Autodesk Fusion 360 part; units mm, degrees
(part 3 of 5)
sketch "Left Projection" plane through (0, 0, 0) normal (0, 0, 1) x (1, 0, 0) in component "Left"
  line L0 (-300.4387, -28.095) -> (-302, -28.095)
  line L1 (-302, -37.905) -> (-300.4387, -37.905)
  arc A0 (-300.4387, -37.905) -> (-298.825, -36.7758) centre (-299.5321, -37.4829) ccw
  line L2 (-298.825, -36.7758) -> (-298.825, -29.2242)
  arc A1 (-298.825, -29.2242) -> (-300.4387, -28.095) centre (-299.5321, -28.5171) ccw
  line L3 (-302, -57.905) -> (-300.4387, -57.905)
  line L4 (-300.4387, -48.095) -> (-302, -48.095)
  arc A2 (-298.825, -49.2242) -> (-300.4387, -48.095) centre (-299.5321, -48.5171) ccw
  line L5 (-298.825, -56.7758) -> (-298.825, -49.2242)
  arc A3 (-300.4387, -57.905) -> (-298.825, -56.7758) centre (-299.5321, -57.4829) ccw
  line L6 (-302, -77.905) -> (-300.4387, -77.905)
  line L7 (-300.4387, -68.095) -> (-302, -68.095)
  arc A4 (-298.825, -69.2242) -> (-300.4387, -68.095) centre (-299.5321, -68.5171) ccw
  line L8 (-298.825, -76.7758) -> (-298.825, -69.2242)
  arc A5 (-300.4387, -77.905) -> (-298.825, -76.7758) centre (-299.5321, -77.4829) ccw
  line L9 (-302, -97.905) -> (-300.4387, -97.905)
  line L10 (-300.4387, -88.095) -> (-302, -88.095)
  arc A6 (-298.825, -89.2242) -> (-300.4387, -88.095) centre (-299.5321, -88.5171) ccw
  line L11 (-298.825, -96.7758) -> (-298.825, -89.2242)
  arc A7 (-300.4387, -97.905) -> (-298.825, -96.7758) centre (-299.5321, -97.4829) ccw
  line L12 (-302, -117.905) -> (-300.4387, -117.905)
  line L13 (-300.4387, -108.095) -> (-302, -108.095)
  arc A8 (-298.825, -109.2242) -> (-300.4387, -108.095) centre (-299.5321, -108.5171) ccw
  line L14 (-298.825, -116.7758) -> (-298.825, -109.2242)
  arc A9 (-300.4387, -117.905) -> (-298.825, -116.7758) centre (-299.5321, -117.4829) ccw
  line L15 (-302, -137.905) -> (-300.4387, -137.905)
  line L16 (-300.4387, -128.095) -> (-302, -128.095)
  arc A10 (-298.825, -129.2242) -> (-300.4387, -128.095) centre (-299.5321, -128.5171) ccw
  line L17 (-298.825, -136.7758) -> (-298.825, -129.2242)
  arc A11 (-300.4387, -137.905) -> (-298.825, -136.7758) centre (-299.5321, -137.4829) ccw
  line L18 (-302, -157.905) -> (-300.4387, -157.905)
  line L19 (-300.4387, -168.095) -> (-302, -168.095)
  arc A12 (-298.825, -169.2242) -> (-300.4387, -168.095) centre (-299.5321, -168.5171) ccw
  line L20 (-298.825, -184) -> (-298.825, -169.2242)
  line L21 (-298.825, -16.7758) -> (-298.825, -2)
  arc A13 (-300.4387, -17.905) -> (-298.825, -16.7758) centre (-299.5321, -17.4829) ccw
  line L22 (-302, -17.905) -> (-300.4387, -17.905)
  line L23 (-300.4387, -148.095) -> (-302, -148.095)
  arc A14 (-298.825, -149.2242) -> (-300.4387, -148.095) centre (-299.5321, -148.5171) ccw
  line L24 (-298.825, -156.7758) -> (-298.825, -149.2242)
  arc A15 (-300.4387, -157.905) -> (-298.825, -156.7758) centre (-299.5321, -157.4829) ccw
  line L25 (-298.825, -2) -> (-286.905, -2)
  line L26 (-286.905, -2) -> (-286.905, -3.5613)
  arc A16 (-286.905, -3.5613) -> (-285.7758, -5.175) centre (-286.4829, -4.4679) ccw
  line L27 (-285.7758, -5.175) -> (-278.2242, -5.175)
  arc A17 (-278.2242, -5.175) -> (-277.095, -3.5613) centre (-277.5171, -4.4679) ccw
  line L28 (-277.095, -3.5613) -> (-277.095, -2)
  line L29 (-277.095, -2) -> (-266.905, -2)
  line L30 (-266.905, -2) -> (-266.905, -3.5613)
  arc A18 (-266.905, -3.5613) -> (-265.7758, -5.175) centre (-266.4829, -4.4679) ccw
  line L31 (-265.7758, -5.175) -> (-258.2242, -5.175)
  arc A19 (-258.2242, -5.175) -> (-257.095, -3.5613) centre (-257.5171, -4.4679) ccw
  line L32 (-257.095, -3.5613) -> (-257.095, -2)
  line L33 (-257.095, -2) -> (-245.175, -2)
  line L34 (-245.175, -2) -> (-245.175, -16.7758)
  arc A20 (-245.175, -16.7758) -> (-243.5613, -17.905) centre (-244.4679, -17.4829) ccw
  line L35 (-243.5613, -17.905) -> (-242, -17.905)
  line L36 (-242, -17.905) -> (-242, -28.095)
  line L37 (-242, -28.095) -> (-243.5613, -28.095)
  arc A21 (-243.5613, -28.095) -> (-245.175, -29.2242) centre (-244.4679, -28.5171) ccw
  line L38 (-245.175, -29.2242) -> (-245.175, -36.7758)
  arc A22 (-245.175, -36.7758) -> (-243.5613, -37.905) centre (-244.4679, -37.4829) ccw
  line L39 (-243.5613, -37.905) -> (-242, -37.905)
  line L40 (-242, -37.905) -> (-242, -48.095)
  line L41 (-243.5613, -48.095) -> (-242, -48.095)
  arc A23 (-243.5613, -48.095) -> (-245.175, -49.2242) centre (-244.4679, -48.5171) ccw
  line L42 (-245.175, -56.7758) -> (-245.175, -49.2242)
  arc A24 (-245.175, -56.7758) -> (-243.5613, -57.905) centre (-244.4679, -57.4829) ccw
  line L43 (-242, -57.905) -> (-243.5613, -57.905)
  line L44 (-242, -57.905) -> (-242, -68.095)
  line L45 (-243.5613, -68.095) -> (-242, -68.095)
  arc A25 (-243.5613, -68.095) -> (-245.175, -69.2242) centre (-244.4679, -68.5171) ccw
  line L46 (-245.175, -76.7758) -> (-245.175, -69.2242)
  arc A26 (-245.175, -76.7758) -> (-243.5613, -77.905) centre (-244.4679, -77.4829) ccw
  line L47 (-242, -77.905) -> (-243.5613, -77.905)
  line L48 (-242, -77.905) -> (-242, -88.095)
  line L49 (-243.5613, -88.095) -> (-242, -88.095)
  arc A27 (-243.5613, -88.095) -> (-245.175, -89.2242) centre (-244.4679, -88.5171) ccw
  line L50 (-245.175, -96.7758) -> (-245.175, -89.2242)
  arc A28 (-245.175, -96.7758) -> (-243.5613, -97.905) centre (-244.4679, -97.4829) ccw
  line L51 (-242, -97.905) -> (-243.5613, -97.905)
  line L52 (-242, -97.905) -> (-242, -108.095)
  line L53 (-243.5613, -108.095) -> (-242, -108.095)
  arc A29 (-243.5613, -108.095) -> (-245.175, -109.2242) centre (-244.4679, -108.5171) ccw
  line L54 (-245.175, -116.7758) -> (-245.175, -109.2242)
  arc A30 (-245.175, -116.7758) -> (-243.5613, -117.905) centre (-244.4679, -117.4829) ccw
  line L55 (-242, -117.905) -> (-243.5613, -117.905)
  line L56 (-242, -117.905) -> (-242, -128.095)
  line L57 (-243.5613, -128.095) -> (-242, -128.095)
  arc A31 (-243.5613, -128.095) -> (-245.175, -129.2242) centre (-244.4679, -128.5171) ccw
  line L58 (-245.175, -136.7758) -> (-245.175, -129.2242)
  arc A32 (-245.175, -136.7758) -> (-243.5613, -137.905) centre (-244.4679, -137.4829) ccw
  line L59 (-242, -137.905) -> (-243.5613, -137.905)
  line L60 (-242, -137.905) -> (-242, -148.095)
  line L61 (-243.5613, -148.095) -> (-242, -148.095)
  arc A33 (-243.5613, -148.095) -> (-245.175, -149.2242) centre (-244.4679, -148.5171) ccw
  line L62 (-245.175, -156.7758) -> (-245.175, -149.2242)
  arc A34 (-245.175, -156.7758) -> (-243.5613, -157.905) centre (-244.4679, -157.4829) ccw
  line L63 (-242, -157.905) -> (-243.5613, -157.905)
  line L64 (-242, -157.905) -> (-242, -168.095)
  line L65 (-243.5613, -168.095) -> (-242, -168.095)
  arc A35 (-243.5613, -168.095) -> (-245.175, -169.2242) centre (-244.4679, -168.5171) ccw
  line L66 (-245.175, -184) -> (-245.175, -169.2242)
  line L67 (-245.175, -184) -> (-257.095, -184)
  line L68 (-257.095, -182.4387) -> (-257.095, -184)
  arc A36 (-257.095, -182.4387) -> (-258.2242, -180.825) centre (-257.5171, -181.5321) ccw
  line L69 (-265.7758, -180.825) -> (-258.2242, -180.825)
  arc A37 (-265.7758, -180.825) -> (-266.905, -182.4387) centre (-266.4829, -181.5321) ccw
  line L70 (-266.905, -184) -> (-266.905, -182.4387)
  line L71 (-266.905, -184) -> (-277.095, -184)
  line L72 (-277.095, -182.4387) -> (-277.095, -184)
  arc A38 (-277.095, -182.4387) -> (-278.2242, -180.825) centre (-277.5171, -181.5321) ccw
  line L73 (-285.7758, -180.825) -> (-278.2242, -180.825)
  arc A39 (-285.7758, -180.825) -> (-286.905, -182.4387) centre (-286.4829, -181.5321) ccw
  line L74 (-286.905, -184) -> (-286.905, -182.4387)
  line L75 (-286.905, -184) -> (-298.825, -184)
  line L76 (-302, -168.095) -> (-302, -157.905)
  line L77 (-302, -148.095) -> (-302, -137.905)
  line L78 (-302, -128.095) -> (-302, -117.905)
  line L79 (-302, -108.095) -> (-302, -97.905)
  line L80 (-302, -88.095) -> (-302, -77.905)
  line L81 (-302, -68.095) -> (-302, -57.905)
  line L82 (-302, -48.095) -> (-302, -37.905)
  line L83 (-302, -28.095) -> (-302, -17.905)
move_body "Move1" [suppressed] in component "Back"
sketch "Back Projection" plane through (0, 0, 0) normal (0, 0, 1) x (1, 0, 0) in component "Back"
  line L0 (5.175, -60.591) -> (5.175, -62.226)
  line L1 (5.175, -62.226) -> (15.7758, -62.226)
  arc A0 (16.905, -63.8397) -> (15.7758, -62.226) centre (16.4829, -62.9331) ccw
  line L2 (16.905, -63.8397) -> (16.905, -65.401)
  line L3 (16.905, -65.401) -> (27.095, -65.401)
  line L4 (27.095, -65.401) -> (27.095, -63.8397)
  arc A1 (28.2242, -62.226) -> (27.095, -63.8397) centre (27.5171, -62.9331) ccw
  line L5 (28.2242, -62.226) -> (35.7758, -62.226)
  arc A2 (36.905, -63.8397) -> (35.7758, -62.226) centre (36.4829, -62.9331) ccw
  line L6 (36.905, -63.8397) -> (36.905, -65.401)
  line L7 (36.905, -65.401) -> (47.095, -65.401)
  line L8 (47.095, -65.401) -> (47.095, -63.8397)
  arc A3 (48.2242, -62.226) -> (47.095, -63.8397) centre (47.5171, -62.9331) ccw
  line L9 (48.2242, -62.226) -> (55.7758, -62.226)
  arc A4 (56.905, -63.8397) -> (55.7758, -62.226) centre (56.4829, -62.9331) ccw
  line L10 (56.905, -63.8397) -> (56.905, -65.401)
  line L11 (56.905, -65.401) -> (67.095, -65.401)
  line L12 (67.095, -65.401) -> (67.095, -63.8397)
  arc A5 (68.2242, -62.226) -> (67.095, -63.8397) centre (67.5171, -62.9331) ccw
  line L13 (68.2242, -62.226) -> (75.7758, -62.226)
  arc A6 (76.905, -63.8397) -> (75.7758, -62.226) centre (76.4829, -62.9331) ccw
  line L14 (76.905, -63.8397) -> (76.905, -65.401)
  line L15 (76.905, -65.401) -> (87.095, -65.401)
  line L16 (87.095, -65.401) -> (87.095, -63.8397)
  arc A7 (88.2242, -62.226) -> (87.095, -63.8397) centre (87.5171, -62.9331) ccw
  line L17 (88.2242, -62.226) -> (95.7758, -62.226)
  arc A8 (96.905, -63.8397) -> (95.7758, -62.226) centre (96.4829, -62.9331) ccw
  line L18 (96.905, -63.8397) -> (96.905, -65.401)
  line L19 (96.905, -65.401) -> (107.095, -65.401)
  line L20 (107.095, -65.401) -> (107.095, -63.8397)
  arc A9 (108.2242, -62.226) -> (107.095, -63.8397) centre (107.5171, -62.9331) ccw
  line L21 (108.2242, -62.226) -> (115.7758, -62.226)
  arc A10 (116.905, -63.8397) -> (115.7758, -62.226) centre (116.4829, -62.9331) ccw
  line L22 (116.905, -63.8397) -> (116.905, -65.401)
  line L23 (116.905, -65.401) -> (127.095, -65.401)
  line L24 (127.095, -65.401) -> (127.095, -63.8397)
  arc A11 (128.2242, -62.226) -> (127.095, -63.8397) centre (127.5171, -62.9331) ccw
  line L25 (128.2242, -62.226) -> (135.7758, -62.226)
  arc A12 (136.905, -63.8397) -> (135.7758, -62.226) centre (136.4829, -62.9331) ccw
  line L26 (136.905, -63.8397) -> (136.905, -65.401)
  line L27 (136.905, -65.401) -> (147.095, -65.401)
  line L28 (147.095, -65.401) -> (147.095, -63.8397)
  arc A13 (148.2242, -62.226) -> (147.095, -63.8397) centre (147.5171, -62.9331) ccw
  line L29 (148.2242, -62.226) -> (155.7758, -62.226)
  arc A14 (156.905, -63.8397) -> (155.7758, -62.226) centre (156.4829, -62.9331) ccw
  line L30 (156.905, -63.8397) -> (156.905, -65.401)
  line L31 (156.905, -65.401) -> (167.095, -65.401)
  line L32 (167.095, -65.401) -> (167.095, -63.8397)
  arc A15 (168.2242, -62.226) -> (167.095, -63.8397) centre (167.5171, -62.9331) ccw
  line L33 (168.2242, -62.226) -> (175.7758, -62.226)
  arc A16 (176.905, -63.8397) -> (175.7758, -62.226) centre (176.4829, -62.9331) ccw
  line L34 (176.905, -63.8397) -> (176.905, -65.401)
  line L35 (176.905, -65.401) -> (187.095, -65.401)
  line L36 (187.095, -65.401) -> (187.095, -63.8397)
  arc A17 (188.2242, -62.226) -> (187.095, -63.8397) centre (187.5171, -62.9331) ccw
  line L37 (188.2242, -62.226) -> (195.7758, -62.226)
  arc A18 (196.905, -63.8397) -> (195.7758, -62.226) centre (196.4829, -62.9331) ccw
  line L38 (196.905, -63.8397) -> (196.905, -65.401)
  line L39 (196.905, -65.401) -> (207.095, -65.401)
  line L40 (207.095, -65.401) -> (207.095, -63.8397)
  arc A19 (208.2242, -62.226) -> (207.095, -63.8397) centre (207.5171, -62.9331) ccw
  line L41 (208.2242, -62.226) -> (215.7758, -62.226)
  arc A20 (216.905, -63.8397) -> (215.7758, -62.226) centre (216.4829, -62.9331) ccw
  line L42 (216.905, -63.8397) -> (216.905, -65.401)
  line L43 (216.905, -65.401) -> (227.095, -65.401)
  line L44 (227.095, -65.401) -> (227.095, -63.8397)
  arc A21 (228.2242, -62.226) -> (227.095, -63.8397) centre (227.5171, -62.9331) ccw
  line L45 (228.2242, -62.226) -> (238.825, -62.226)
  line L46 (238.825, -62.226) -> (238.825, -60.591)
  arc A22 (238.825, -59.1768) -> (238.825, -60.591) centre (239.5321, -59.8839) ccw
  line L47 (238.825, -59.1768) -> (238.825, -51.6252)
  arc A23 (240.4387, -50.496) -> (238.825, -51.6252) centre (239.5321, -50.9181) ccw
  line L48 (240.4387, -50.496) -> (242, -50.496)
  line L49 (242, -50.496) -> (242, -40.306)
  line L50 (242, -40.306) -> (240.4387, -40.306)
  arc A24 (238.825, -39.1768) -> (240.4387, -40.306) centre (239.5321, -39.8839) ccw
  line L51 (238.825, -39.1768) -> (238.825, -31.6252)
  arc A25 (240.4387, -30.496) -> (238.825, -31.6252) centre (239.5321, -30.9181) ccw
  line L52 (240.4387, -30.496) -> (242, -30.496)
  line L53 (242, -30.496) -> (242, -20.306)
  line L54 (242, -20.306) -> (240.4387, -20.306)
  arc A26 (238.825, -19.1768) -> (240.4387, -20.306) centre (239.5321, -19.8839) ccw
  line L55 (238.825, -19.1768) -> (238.825, -11.6252)
  arc A27 (238.825, -10.211) -> (238.825, -11.6252) centre (239.5321, -10.9181) ccw
  line L56 (238.825, -10.211) -> (238.825, -8.576)
  line L57 (238.825, -8.576) -> (228.2242, -8.576)
  arc A28 (227.095, -6.9623) -> (228.2242, -8.576) centre (227.5171, -7.8689) ccw
  line L58 (227.095, -6.9623) -> (227.095, -5.401)
  line L59 (227.095, -5.401) -> (216.905, -5.401)
  line L60 (216.905, -5.401) -> (216.905, -6.9623)
  arc A29 (215.7758, -8.576) -> (216.905, -6.9623) centre (216.4829, -7.8689) ccw
  line L61 (215.7758, -8.576) -> (208.2242, -8.576)
  arc A30 (207.095, -6.9623) -> (208.2242, -8.576) centre (207.5171, -7.8689) ccw
  line L62 (207.095, -6.9623) -> (207.095, -5.401)
  line L63 (207.095, -5.401) -> (196.905, -5.401)
  line L64 (196.905, -5.401) -> (196.905, -6.9623)
  arc A31 (195.7758, -8.576) -> (196.905, -6.9623) centre (196.4829, -7.8689) ccw
  line L65 (195.7758, -8.576) -> (188.2242, -8.576)
  arc A32 (187.095, -6.9623) -> (188.2242, -8.576) centre (187.5171, -7.8689) ccw
  line L66 (187.095, -6.9623) -> (187.095, -5.401)
  line L67 (187.095, -5.401) -> (176.905, -5.401)
  line L68 (176.905, -5.401) -> (176.905, -6.9623)
  arc A33 (175.7758, -8.576) -> (176.905, -6.9623) centre (176.4829, -7.8689) ccw
  line L69 (175.7758, -8.576) -> (168.2242, -8.576)
  arc A34 (167.095, -6.9623) -> (168.2242, -8.576) centre (167.5171, -7.8689) ccw
  line L70 (167.095, -6.9623) -> (167.095, -5.401)
  line L71 (167.095, -5.401) -> (156.905, -5.401)
  line L72 (156.905, -5.401) -> (156.905, -6.9623)
  arc A35 (155.7758, -8.576) -> (156.905, -6.9623) centre (156.4829, -7.8689) ccw
  line L73 (155.7758, -8.576) -> (148.2242, -8.576)
  arc A36 (147.095, -6.9623) -> (148.2242, -8.576) centre (147.5171, -7.8689) ccw
  line L74 (147.095, -6.9623) -> (147.095, -5.401)
  line L75 (147.095, -5.401) -> (136.905, -5.401)
  line L76 (136.905, -5.401) -> (136.905, -6.9623)
  arc A37 (135.7758, -8.576) -> (136.905, -6.9623) centre (136.4829, -7.8689) ccw
  line L77 (135.7758, -8.576) -> (128.2242, -8.576)
  arc A38 (127.095, -6.9623) -> (128.2242, -8.576) centre (127.5171, -7.8689) ccw
  line L78 (127.095, -6.9623) -> (127.095, -5.401)
  line L79 (127.095, -5.401) -> (116.905, -5.401)
  line L80 (116.905, -5.401) -> (116.905, -6.9623)
  arc A39 (115.7758, -8.576) -> (116.905, -6.9623) centre (116.4829, -7.8689) ccw
  line L81 (115.7758, -8.576) -> (108.2242, -8.576)
  arc A40 (107.095, -6.9623) -> (108.2242, -8.576) centre (107.5171, -7.8689) ccw
  line L82 (107.095, -6.9623) -> (107.095, -5.401)
  line L83 (107.095, -5.401) -> (96.905, -5.401)
  line L84 (96.905, -5.401) -> (96.905, -6.9623)
  arc A41 (95.7758, -8.576) -> (96.905, -6.9623) centre (96.4829, -7.8689) ccw
  line L85 (95.7758, -8.576) -> (88.2242, -8.576)
  arc A42 (87.095, -6.9623) -> (88.2242, -8.576) centre (87.5171, -7.8689) ccw
  line L86 (87.095, -6.9623) -> (87.095, -5.401)
  line L87 (87.095, -5.401) -> (76.905, -5.401)
  line L88 (76.905, -5.401) -> (76.905, -6.9623)
  arc A43 (75.7758, -8.576) -> (76.905, -6.9623) centre (76.4829, -7.8689) ccw
  line L89 (75.7758, -8.576) -> (68.2242, -8.576)
  arc A44 (67.095, -6.9623) -> (68.2242, -8.576) centre (67.5171, -7.8689) ccw
  line L90 (67.095, -6.9623) -> (67.095, -5.401)
  line L91 (67.095, -5.401) -> (56.905, -5.401)
  line L92 (56.905, -5.401) -> (56.905, -6.9623)
  arc A45 (55.7758, -8.576) -> (56.905, -6.9623) centre (56.4829, -7.8689) ccw
  line L93 (55.7758, -8.576) -> (48.2242, -8.576)
  arc A46 (47.095, -6.9623) -> (48.2242, -8.576) centre (47.5171, -7.8689) ccw
  line L94 (47.095, -6.9623) -> (47.095, -5.401)
  line L95 (47.095, -5.401) -> (36.905, -5.401)
  line L96 (36.905, -5.401) -> (36.905, -6.9623)
  arc A47 (35.7758, -8.576) -> (36.905, -6.9623) centre (36.4829, -7.8689) ccw
  line L97 (35.7758, -8.576) -> (28.2242, -8.576)
  arc A48 (27.095, -6.9623) -> (28.2242, -8.576) centre (27.5171, -7.8689) ccw
  line L98 (27.095, -6.9623) -> (27.095, -5.401)
  line L99 (27.095, -5.401) -> (16.905, -5.401)
  line L100 (16.905, -5.401) -> (16.905, -6.9623)
  arc A49 (15.7758, -8.576) -> (16.905, -6.9623) centre (16.4829, -7.8689) ccw
  line L101 (15.7758, -8.576) -> (5.175, -8.576)
  line L102 (5.175, -8.576) -> (5.175, -10.211)
  arc A50 (5.175, -11.6252) -> (5.175, -10.211) centre (4.4679, -10.9181) ccw
  line L103 (5.175, -11.6252) -> (5.175, -19.1768)
  arc A51 (3.5613, -20.306) -> (5.175, -19.1768) centre (4.4679, -19.8839) ccw
  line L104 (3.5613, -20.306) -> (2, -20.306)
  line L105 (2, -20.306) -> (2, -30.496)
  line L106 (2, -30.496) -> (3.5613, -30.496)
  arc A52 (5.175, -31.6252) -> (3.5613, -30.496) centre (4.4679, -30.9181) ccw
  line L107 (5.175, -31.6252) -> (5.175, -39.1768)
  arc A53 (3.5613, -40.306) -> (5.175, -39.1768) centre (4.4679, -39.8839) ccw
  line L108 (3.5613, -40.306) -> (2, -40.306)
  line L109 (2, -40.306) -> (2, -50.496)
  line L110 (2, -50.496) -> (3.5613, -50.496)
  arc A54 (5.175, -51.6252) -> (3.5613, -50.496) centre (4.4679, -50.9181) ccw
  line L111 (5.175, -51.6252) -> (5.175, -59.1768)
  arc A55 (5.175, -60.591) -> (5.175, -59.1768) centre (4.4679, -59.8839) ccw
sketch "Plaform" plane through (0, 0, 0) normal (0, 0, 1) x (1, 0, 0) in component "Platform"
  line L0 (-255.6038, 317) -> (-88.6038, 317)
  line L1 (-85.6038, 314) -> (-85.6038, 203)
  line L2 (-88.6038, 200) -> (-255.6038, 200)
  line L3 (-258.6038, 203) -> (-258.6038, 314)
  line L4 (1.75, 0) -> (22.5, 0)
  line L5 (0, 1.75) -> (0, 22.5)
  line L6 (-178.6038, 263) -> (-165.6038, 263)
  line L7 (-163.6038, 261) -> (-163.6038, 256)
  line L8 (-165.6038, 254) -> (-178.6038, 254)
  line L9 (-180.6038, 256) -> (-180.6038, 261)
  line L10 (-187.1038, 314) -> (-157.1038, 314) construction
  line L11 (-157.1038, 314) -> (-157.1038, 203) construction
  line L12 (-157.1038, 203) -> (-187.1038, 203) construction
  line L13 (-187.1038, 203) -> (-187.1038, 314) construction
  line L14 (-187.1038, 314) -> (-157.1038, 203) construction
  line L15 (-157.1038, 314) -> (-187.1038, 203) construction
  circle A0 centre (-187.1038, 314) radius 1.5
  circle A1 centre (-157.1038, 314) radius 1.5
  circle A2 centre (-157.1038, 203) radius 1.5
  circle A3 centre (-187.1038, 203) radius 1.5
  line L16 (-239.1038, 305) -> (-105.1038, 305) construction
  line L17 (-105.1038, 212) -> (-239.1038, 212) construction
  line L18 (-239.1038, 212) -> (-239.1038, 305) construction
  line L19 (-239.1038, 305) -> (-105.1038, 212) construction
  line L20 (-105.1038, 305) -> (-239.1038, 212) construction
  line L21 (-89.1038, 203.5) -> (-255.1038, 203.5) construction
  line L22 (-255.1038, 203.5) -> (-255.1038, 313.5) construction
  line L23 (-255.1038, 313.5) -> (-89.1038, 313.5) construction
  line L24 (-89.1038, 203.5) -> (-255.1038, 313.5) construction
  line L25 (-255.1038, 203.5) -> (-89.1038, 313.5) construction
  circle A4 centre (-255.1038, 203.5) radius 1.75
  circle A5 centre (-255.1038, 313.5) radius 1.75
  circle A6 centre (-89.1038, 313.5) radius 1.75
  circle A7 centre (-89.1038, 203.5) radius 1.75
  circle A8 centre (-118.6038, 258.5) radius 1.5
  circle A9 centre (-88.6038, 258.5) radius 1.5
  arc A10 (-88.6038, 200) -> (-85.6038, 203) centre (-88.6038, 203) ccw
  arc A11 (-258.6038, 203) -> (-255.6038, 200) centre (-255.6038, 203) ccw
  arc A12 (-255.6038, 317) -> (-258.6038, 314) centre (-255.6038, 314) ccw
  arc A13 (-85.6038, 314) -> (-88.6038, 317) centre (-88.6038, 314) ccw
  circle A14 centre (-239.1038, 305) radius 1.75
  circle A15 centre (-105.1038, 305) radius 1.75
  circle A16 centre (-105.1038, 212) radius 1.75
  circle A17 centre (-239.1038, 212) radius 1.75
  line L26 (-105.1038, 305) -> (-105.1038, 212) construction
  arc A18 (-178.6038, 263) -> (-180.6038, 261) centre (-178.6038, 261) ccw
  arc A19 (-163.6038, 261) -> (-165.6038, 263) centre (-165.6038, 261) ccw
  arc A20 (-180.6038, 256) -> (-178.6038, 254) centre (-178.6038, 256) ccw
  arc A21 (-165.6038, 254) -> (-163.6038, 256) centre (-165.6038, 256) ccw
  point P0 (-258.6038, 317)
  point P1 (-85.6038, 317)
  point P2 (-258.6038, 200)
  point P3 (-180.6038, 263)
  point P4 (-163.6038, 263)
  point P5 (-180.6038, 254)
  point P6 (-85.6038, 258.5)
  point P7 (-172.1038, 263)
  point P8 (-172.1038, 317)
  point P9 (-172.1038, 258.5)
  point P10 (-172.1038, 258.5)
  point P11 (-172.1038, 258.5)
  point P12 (-258.6038, 258.5)
  point P13 (-172.1038, 200)
  point P14 (-255.1038, 258.5)
  point P15 (-180.6038, 258.5)
  point P16 (-172.1038, 254)
  dimension "d1498" = 173
  dimension "d1499" = 117
  dimension "d1500" = 200
  dimension "d1501" = 85.6038
  dimension "d1502" = 17
  dimension "d1503" = 9
  dimension "d1505" = 30
  dimension "d1506" = 111
  dimension "d1507" = 3
  dimension "d1508" = 3
  dimension "d1509" = 3
  dimension "d1510" = 3
  dimension "d1512" = 93
  dimension "d1513" = 166
  dimension "d1514" = 110
  dimension "d1515" = 3.5
  dimension "d1516" = 3.5
  dimension "d1517" = 3.5
  dimension "d1518" = 3.5
  dimension "d1552" = 3
  dimension "d1553" = 3
  dimension "d1554" = 3
  dimension "d1555" = 3
  dimension "d1557" = 3.5
  dimension "d1558" = 3.5
  dimension "d1559" = 3.5
  dimension "d1560" = 3.5
  dimension "d1611" = 3
  dimension "d1612" = 3
  dimension "d1613" = 3
  dimension "d1614" = 30
  dimension "d1615" = 134
  dimension "d1650" = 2
  dimension "d1651" = 2
  dimension "d1652" = 2
  dimension "d1653" = 2
  dimension "d1736" = 9
  constraint horizontal L0
  constraint vertical L1
  constraint horizontal L2
  constraint vertical L3
  constraint horizontal L6
  constraint vertical L7
  constraint horizontal L8
  constraint vertical L9
  constraint vertical P7 P8
  constraint horizontal L10
  constraint perpendicular L10 L11
  constraint parallel L10 L12
  constraint parallel L11 L13
  constraint coincident L14 P11
  constraint coincident L15 P11
  constraint horizontal P6 P10
  constraint vertical P8 P11
  constraint coincident L10.start L13.end
  constraint coincident L10.end L11.start
  constraint coincident L11.end L12.start
  constraint coincident L12.end L13.start
  constraint horizontal L16
  constraint parallel L16 L17
  constraint coincident L19 P11
  constraint coincident L20 P11
  constraint coincident P11 P10
  constraint horizontal L21
  constraint perpendicular L21 L22
  constraint parallel L21 L23
  constraint coincident L24 P11
  constraint coincident L25 P11
  constraint coincident L21.end L22.start
  constraint coincident L22.end L23.start
  constraint coincident L23.end L25.end
  constraint coincident L21.start L24.start
  constraint coincident L1 P6
  constraint tangent L2 A10
  constraint tangent L1 A10
  constraint coincident P2 L2
  constraint coincident P2 L3
  constraint tangent L2 A11
  constraint tangent L3 A11
  constraint coincident L0 P8
  constraint coincident P0 L3
  constraint coincident P0 L0
  constraint tangent L3 A12
  constraint tangent L0 A12
  constraint midpoint L3 P12
  constraint horizontal P11 P12
  constraint midpoint L2 P13
  constraint vertical P11 P13
  constraint coincident P1 L0
  constraint coincident P1 L1
  constraint tangent L0 A13
  constraint tangent L1 A13
  constraint coincident L16.start L18.end
  constraint coincident L16.end L20.start
  constraint coincident L17.start L19.end
  constraint coincident L17.end L18.start
  constraint perpendicular L17 L26
  constraint perpendicular L17 L18
  constraint horizontal A8.centre A9.centre
  constraint horizontal P6 A9.centre
  constraint midpoint L22 P14
  constraint horizontal P12 P14
  constraint coincident L6 P7
  constraint coincident P3 L9
  constraint coincident P3 L6
  constraint tangent L9 A18
  constraint tangent L6 A18
  constraint coincident P4 L6
  constraint coincident P4 L7
  constraint tangent L6 A19
  constraint tangent L7 A19
  constraint coincident P5 L9
  constraint coincident P5 L8
  constraint tangent L9 A20
  constraint tangent L8 A20
  constraint tangent L8 A21
  constraint tangent L7 A21
  constraint midpoint L9 P15
  constraint horizontal P11 P15
  constraint midpoint L8 P16
  constraint vertical P11 P16
  measures "d1498" distance of P0 P1
  measures "d1499" distance of P0 P2
  measures "d1500" distance of L2 L4
  measures "d1501" distance of L1 L5
  measures "d1502" distance of P3 P4
  measures "d1503" distance of P3 P5
  measures "d1505" distance of L11.end L12.end
  measures "d1506" distance of L10.start L12.end
  measures "d1507" diameter of A0
  measures "d1508" diameter of A1
  measures "d1509" diameter of A2
  measures "d1510" diameter of A3
  measures "d1512" distance of L16 L17
  measures "d1513" distance of L22.end L23.end
  measures "d1514" distance of L21.end L22.end
  measures "d1515" diameter of A4
  measures "d1516" diameter of A5
  measures "d1517" diameter of A6
  measures "d1518" diameter of A7
  measures "d1552" radius of A10
  measures "d1553" radius of A11
  measures "d1554" radius of A12
  measures "d1555" radius of A13
  measures "d1557" diameter of A14
  measures "d1558" diameter of A15
  measures "d1559" diameter of A16
  measures "d1560" diameter of A17
  measures "d1611" distance of L1 A9.centre
  measures "d1612" diameter of A8
  measures "d1613" diameter of A9
  measures "d1614" distance of A8.centre A9.centre
  measures "d1615" distance of L17.start L17.end
  measures "d1650" radius of A18
  measures "d1651" radius of A19
  measures "d1652" radius of A20
  measures "d1653" radius of A21
  measures "d1736" distance of L6 L8
extrude "Extrude1" [suppressed] in component "Platform"
copy_body "CopyPasteBodies12" [suppressed]
move_body "Move37" [suppressed]
copy_body "Body->Comp12" [suppressed] in component "Brace"
sketch "Contents" plane through (0, 0, 0) normal (0, 0, 1) x (1, 0, 0) in component "Brace"
  circle A0 centre (34, 34.6) radius 15
  line L0 (40, 122) -> (22, 122)
  line L1 (60, 0) -> (0, 0) construction
  line L2 (18.5, 19.1) -> (18.5, 50.1) construction
  circle A1 centre (53, 31) radius 1.25
  circle A2 centre (53, 61) radius 1.25
  circle A3 centre (53, 121) radius 1.25
  line L3 (0, 0) -> (0, 182) construction
  line L4 (49.5, 19.1) -> (18.5, 50.1) construction
  circle A4 centre (18.5, 50.1) radius 1.5
  circle A5 centre (53, 91) radius 1.25
  line L5 (49.5, 50.1) -> (49.5, 19.1) construction
  line L6 (22, 162) -> (40, 162)
  line L7 (18.5, 19.1) -> (49.5, 50.1) construction
  circle A6 centre (53, 151) radius 1.25
  circle A7 centre (49.5, 19.1) radius 1.5
  line L8 (18.5, 50.1) -> (49.5, 50.1) construction
  line L9 (49.5, 19.1) -> (18.5, 19.1) construction
  line L10 (0, 182) -> (60, 182) construction
  circle A8 centre (18.5, 19.1) radius 1.5
  circle A9 centre (49.5, 50.1) radius 1.5
  line L11 (40, 162) -> (40, 122)
  line L12 (60, 182) -> (60, 0) construction
  line L13 (3.175, 95) -> (13.175, 95)
  line L14 (13.175, 95) -> (13.175, 87)
  line L15 (13.175, 87) -> (3.175, 87)
  line L16 (0, 425.6) -> (0, -184)
  line L17 (27.6442, 147.907) -> (28.3894, 146.7583)
  line L18 (34.519, 148.0232) -> (33.9924, 147.4295)
  arc A10 (33.9924, 147.4295) -> (27.6442, 147.907) centre (31, 150.0839) ccw
  line L19 (32, 141.3873) -> (32, 132.9489)
  line L20 (30, 132.9489) -> (30, 141.316)
  line L21 (31.1201, 154.0821) -> (30.7651, 146.624) construction
  line L22 (30, 132.9489) -> (32, 132.9489)
  arc A11 (34.519, 148.0232) -> (32, 141.3873) centre (42, 141.3873) ccw
  arc A12 (30, 141.316) -> (28.3894, 146.7583) centre (20, 141.316) ccw
  line L23 (31, 150.0839) -> (31, 109.1329) construction
  line L24 (19.1457, 161.9685) -> (15.5387, 161.9685)
  line L25 (15.5387, 161.9685) -> (15.5387, 153.7089)
  line L26 (19.1457, 161.1035) -> (22, 161.1035)
  line L27 (22, 158.4561) -> (22, 154.2014)
  line L28 (19.1457, 157.1289) -> (19.1457, 158.4561)
  line L29 (19.1457, 158.4561) -> (22, 158.4561)
  line L30 (22, 158.4561) -> (22, 157.1289)
  line L31 (19.1457, 153.7089) -> (19.1457, 158.4561)
  line L32 (19.1457, 161.1035) -> (19.1457, 161.9685)
  line L33 (15.5387, 153.7089) -> (19.1457, 153.7089)
  line L34 (22, 122) -> (22, 158.4561)
  line L35 (22, 161.1035) -> (22, 162)
  point P0 (60, 91)
  point P1 (34, 34.6)
  point P2 (0, 182)
  dimension "d1134" = 33
  dimension "d1135" = -30
  dimension "d1136" = 182
  dimension "d1137" = 60
  dimension "d974" = 2.5
  dimension "d975" = 7
  dimension "d1140" = 31
  dimension "d1141" = 31
  dimension "d1142" = 30
  dimension "d1143" = 3
  dimension "d1144" = 3
  dimension "d1145" = 3
  dimension "d1146" = 3
  dimension "d1147" = 26
  dimension "d1148" = 34.6
  dimension "d1149" = 20
  dimension "d1011" = 20
  dimension "d1012" = 18
  dimension "d1013" = 40
  dimension "d1716" = 3.175
  dimension "d1717" = 8
  dimension "d1718" = 87
  dimension "d1719" = 10
  dimension "d1720" = 9
  dimension "d1721" = 8
  dimension "d1722" = 2
  dimension "d1723" = 10
  dimension "d1724" = 10
  constraint perpendicular L1 L12
  constraint parallel L3 L12
  constraint coincident P2 L3.end
  constraint perpendicular L10 L12
  constraint midpoint P0 L12
  constraint horizontal P0 A5.centre
  constraint horizontal L9
  constraint perpendicular L2 L9
  constraint parallel L8 L9
  constraint parallel L2 L5
  constraint coincident P1 L4
  constraint coincident P1 L7
  constraint coincident P1 A0.centre
  constraint coincident L2.end L4.end
  constraint coincident L5.start L7.end
  constraint coincident L4.start L5.end
  constraint coincident L2.start L7.start
  constraint horizontal L6
  constraint vertical L11
  constraint horizontal L0
  constraint vertical L34
  constraint coincident L1.end L3.start
  constraint horizontal L13
  constraint vertical L14
  constraint horizontal L15
  constraint tangent L18 A10
  constraint tangent L17 A10
  constraint parallel L19 L20
  constraint coincident A10 L21.start
  constraint horizontal L22
  constraint tangent L18 A11
  constraint tangent L19 A11
  constraint tangent L17 A12
  constraint tangent L20 A12
  constraint coincident A10.centre L23.start
  constraint perpendicular L0 L23
  constraint horizontal L24
  constraint vertical L25
  constraint vertical L31
  constraint horizontal L26
  constraint vertical L27
  constraint coincident L27.end L34
  constraint coincident L26.start L31
  constraint vertical L28
  constraint horizontal L29
  constraint vertical L30
  constraint coincident L30.end L34
  constraint collinear L31 L32
  constraint perpendicular L31 L33
  constraint coincident L26.end L34
  constraint collinear L34 L35
  measures "d1136" distance of L1.end P2
  measures "d1137" distance of L1.end L1.start
  measures "d974" diameter of A5
  measures "d975" distance of A5.centre L12
  measures "d1140" distance of L2.end L5.start
  measures "d1141" distance of L2.end L2.start
  measures "d1142" diameter of A0
  measures "d1143" diameter of A4
  measures "d1144" diameter of A9
  measures "d1145" diameter of A7
  measures "d1146" diameter of A8
  measures "d1147" distance of P1 L12
  measures "d1148" distance of P1 L1
  measures "d1149" distance of L6.start L10
  measures "d1011" distance of L11 L12
  measures "d1012" distance of L0.end L0.start
  measures "d1013" distance of L0.end L6.start
  measures "d1716" distance of L13.start L16
  measures "d1717" distance of L13.end L14.end
  measures "d1718" distance of L10 L13
  measures "d1719" distance of L13.start L13.end
  measures "d1720" distance of A10.centre L34
  measures "d1721" diameter of A10
  measures "d1722" distance of L19.end L20.start
  measures "d1723" radius of A11
  measures "d1724" radius of A12
sketch "Content" plane through (0, 0, 0) normal (0, 0, 1) x (1, 0, 0) in component "Top"
  line L0 (-132, 172) -> (-116, 172)
  circle A0 centre (-49, 80) radius 1.5
  circle A1 centre (-49, 102) radius 1.5
  line L1 (0, 0) -> (-240, 0) construction
  line L2 (-114, 170) -> (-114, 127.9999)
  line L3 (-240, 182) -> (0, 182) construction
  line L4 (0, 182) -> (0, 0) construction
  circle A2 centre (-58, 151) radius 1.5
  circle A3 centre (-53, 136) radius 1.5
  circle A4 centre (-48, 151) radius 1.5
  circle A5 centre (-68, 146) radius 1.5
  circle A6 centre (-48, 146) radius 1.5
  circle A7 centre (-48, 156) radius 1.5
  circle A8 centre (-58, 156) radius 1.5
  circle A9 centre (-63, 141) radius 1.5
  circle A10 centre (-63, 151) radius 1.5
  circle A11 centre (-63, 146) radius 1.5
  circle A12 centre (-48, 141) radius 1.5
  circle A13 centre (-58, 146) radius 1.5
  circle A14 centre (-68, 151) radius 1.5
  line L5 (-163.976, 90) -> (-163.976, 96)
  circle A15 centre (-68, 136) radius 1.5
  circle A16 centre (-63, 156) radius 1.5
  circle A17 centre (-68, 156) radius 1.5
  circle A18 centre (-48, 136) radius 1.5
  circle A19 centre (-58, 136) radius 1.5
  line L6 (-240, 0) -> (-240, 182) construction
  circle A20 centre (-191, 102) radius 1.5
  circle A21 centre (-53, 156) radius 1.5
  circle A22 centre (-191, 80) radius 1.5
  line L7 (-134, 128) -> (-134, 170)
  circle A23 centre (-53, 146) radius 1.5
  line L8 (-159.976, 88) -> (-161.976, 88)
  line L9 (-161.976, 98) -> (-159.976, 98)
  circle A24 centre (-63, 136) radius 1.5
  line L10 (-157.976, 96) -> (-157.976, 90)
  circle A25 centre (-53, 141) radius 1.5
  circle A26 centre (-58, 141) radius 1.5
  circle A27 centre (-53, 151) radius 1.5
  line L11 (-116, 125.9999) -> (-132, 126)
  circle A28 centre (-68, 141) radius 1.5
  line L12 (0, 1.75) -> (0, 22.5)
  line L13 (1.75, 0) -> (22.5, 0)
  circle A29 centre (-68, 131) radius 1.5
  circle A30 centre (-63, 131) radius 1.5
  circle A31 centre (-58, 131) radius 1.5
  circle A32 centre (-53, 131) radius 1.5
  circle A33 centre (-48, 131) radius 1.5
  arc A34 (-161.976, 98) -> (-163.976, 96) centre (-161.976, 96) ccw
  arc A35 (-163.976, 90) -> (-161.976, 88) centre (-161.976, 90) ccw
  arc A36 (-159.976, 88) -> (-157.976, 90) centre (-159.976, 90) ccw
  arc A37 (-157.976, 96) -> (-159.976, 98) centre (-159.976, 96) ccw
  arc A38 (-132, 172) -> (-134, 170) centre (-132, 170) ccw
  arc A39 (-114, 170) -> (-116, 172) centre (-116, 170) ccw
  arc A40 (-116, 125.9999) -> (-114, 127.9999) centre (-116, 127.9999) ccw
  arc A41 (-134, 128) -> (-132, 126) centre (-132, 128) ccw
  line L14 (-131.3, 149.5) -> (-115.3, 149.5)
  circle A42 centre (-47, 47) radius 1.5
  circle A43 centre (-37, 62) radius 1.5
  circle A44 centre (-52, 47) radius 1.5
  circle A45 centre (-57, 67) radius 1.5
  circle A46 centre (-57, 57) radius 1.5
  circle A47 centre (-47, 67) radius 1.5
  circle A48 centre (-52, 57) radius 1.5
  circle A49 centre (-57, 47) radius 1.5
  circle A50 centre (-42, 62) radius 1.5
  circle A51 centre (-52, 52) radius 1.5
  circle A52 centre (-47, 62) radius 1.5
  circle A53 centre (-37, 52) radius 1.5
  circle A54 centre (-47, 52) radius 1.5
  circle A55 centre (-57, 62) radius 1.5
  circle A56 centre (-47, 57) radius 1.5
  circle A57 centre (-52, 67) radius 1.5
  circle A58 centre (-42, 52) radius 1.5
  circle A59 centre (-42, 57) radius 1.5
  circle A60 centre (-57, 52) radius 1.5
  circle A61 centre (-42, 47) radius 1.5
  circle A62 centre (-37, 67) radius 1.5
  circle A63 centre (-52, 62) radius 1.5
  circle A64 centre (-42, 67) radius 1.5
  circle A65 centre (-37, 57) radius 1.5
  circle A66 centre (-37, 47) radius 1.5
  line L15 (-242, 182) -> (-242, 0)
  circle A67 centre (-57, 42) radius 1.5
  circle A68 centre (-52, 42) radius 1.5
  circle A69 centre (-47, 42) radius 1.5
  circle A70 centre (-42, 42) radius 1.5
  circle A71 centre (-37, 42) radius 1.5
  circle A72 centre (-210, 15) radius 1.5
  circle A73 centre (-215, 30) radius 1.5
  circle A74 centre (-205, 25) radius 1.5
  circle A75 centre (-205, 30) radius 1.5
  circle A76 centre (-195, 20) radius 1.5
  circle A77 centre (-200, 30) radius 1.5
  circle A78 centre (-210, 20) radius 1.5
  circle A79 centre (-205, 15) radius 1.5
  circle A80 centre (-210, 30) radius 1.5
  circle A81 centre (-210, 10) radius 1.5
  circle A82 centre (-200, 10) radius 1.5
  circle A83 centre (-210, 25) radius 1.5
  circle A84 centre (-215, 25) radius 1.5
  circle A85 centre (-215, 15) radius 1.5
  circle A86 centre (-200, 25) radius 1.5
  circle A87 centre (-200, 20) radius 1.5
  circle A88 centre (-215, 10) radius 1.5
  circle A89 centre (-215, 20) radius 1.5
  circle A90 centre (-205, 10) radius 1.5
  circle A91 centre (-195, 10) radius 1.5
  circle A92 centre (-195, 25) radius 1.5
  circle A93 centre (-205, 20) radius 1.5
  circle A94 centre (-195, 15) radius 1.5
  circle A95 centre (-195, 30) radius 1.5
  circle A96 centre (-200, 15) radius 1.5
  line L16 (-240, 0) -> (-240, 182)
  circle A97 centre (-128.0762, 158.5418) radius 1.6
  circle A98 centre (-128.0762, 158.5418) radius 3.5
  circle A99 centre (-119.0762, 158.5418) radius 1.6
  circle A100 centre (-119.0762, 158.5418) radius 3.5
  circle A101 centre (-128.0762, 167.5418) radius 1.6
  circle A102 centre (-128.0762, 167.5418) radius 3.5
  circle A103 centre (-119.0762, 167.5418) radius 1.6
  circle A104 centre (-119.0762, 167.5418) radius 3.5
  arc A105 (-124.6, 139.8073) -> (-127.2667, 146.606) centre (-134.6, 139.8073) ccw
  line L17 (-124.6, 128.3707) -> (-122.8, 152.6283) construction
  arc A106 (-119.9333, 146.606) -> (-122.6, 139.8073) centre (-112.6, 139.8073) ccw
  line L18 (-124.6, 128.3707) -> (-124.6, 139.8073)
  line L19 (-122.6, 128.3707) -> (-124.6, 128.3707)
  line L20 (-122.6, 128.3707) -> (-124.6, 152.6283) construction
  line L21 (-122.6, 139.8073) -> (-122.6, 128.3707)
  arc A107 (-119.9333, 146.606) -> (-127.2667, 146.606) centre (-123.6, 150.0053) ccw
  point P0 (-134, 172)
  point P1 (-160.976, 126.0001)
  point P2 (-157.976, 98)
  point P3 (-114, 172)
  point P4 (-134, 126)
  point P5 (-160.976, 98)
  point P6 (-163.976, 98)
  point P7 (-163.976, 88)
  point P8 (-123.6526, 141.1379)
  dimension "d1161" = 142
  dimension "d1163" = 240
  dimension "d1164" = 182
  dimension "d1165" = 20
  dimension "d1166" = 46
  dimension "d1167" = 6
  dimension "d1168" = 10
  dimension "d1169" = 10
  dimension "d1170" = 106
  dimension "d1171" = 84
  dimension "d1172" = 26
  dimension "d1173" = 3
  dimension "d1174" = 68
  dimension "d1175" = 3
  dimension "d1176" = 49
  dimension "d1177" = 80
  dimension "d1600" = 2
  dimension "d1601" = 2
  dimension "d1602" = 2
  dimension "d1603" = 2
  dimension "d1604" = 2
  dimension "d1605" = 2
  dimension "d1606" = 2
  dimension "d1607" = 2
  dimension "d1696" = 3
  dimension "d1699" = 47
  dimension "d1700" = 47
  dimension "d1705" = 3
  dimension "d1707" = 30
  dimension "d1708" = 20
  dimension "d1709" = 3.2
  dimension "d1710" = 7
  dimension "d1713" = 9
  dimension "d1714" = 9
  dimension "d1739" = 1.8
  dimension "d1740" = 10
  dimension "d1741" = 10
  dimension "d1742" = 10
  constraint horizontal L3
  constraint perpendicular L3 L4
  constraint horizontal L0
  constraint vertical L2
  constraint vertical L7
  constraint horizontal L9
  constraint vertical L10
  constraint horizontal L8
  constraint vertical L5
  constraint vertical P1 P5
  constraint perpendicular L1 L6
  constraint collinear L4 L12
  constraint collinear L1 L13
  constraint coincident P5 L9
  constraint coincident P6 L9
  constraint coincident P6 L5
  constraint tangent L9 A34
  constraint tangent L5 A34
  constraint coincident P7 L8
  constraint coincident P7 L5
  constraint tangent L8 A35
  constraint tangent L5 A35
  constraint tangent L8 A36
  constraint tangent L10 A36
  constraint coincident P2 L10
  constraint coincident P2 L9
  constraint tangent L10 A37
  constraint tangent L9 A37
  constraint coincident P0 L0
  constraint coincident P0 L7
  constraint tangent L0 A38
  constraint tangent L7 A38
  constraint coincident P3 L0
  constraint coincident P3 L2
  constraint tangent L0 A39
  constraint tangent L2 A39
  constraint coincident P1 L11
  constraint tangent L11 A40
  constraint tangent L2 A40
  constraint coincident P4 L7
  constraint coincident P4 L11
  constraint tangent L7 A41
  constraint tangent L11 A41
  constraint equal L0 L11
  constraint midpoint P5 L9
  constraint concentric A97 A98
  constraint horizontal L19
  constraint perpendicular L18 L19
  constraint parallel L18 L21
  constraint coincident P8 L20
  constraint coincident P8 L17
  constraint tangent A106 A107
  constraint tangent A106 L21
  constraint tangent A105 A107
  constraint tangent A105 L18
  measures "d1163" distance of L3.end L3.start
  measures "d1164" distance of L1.end L3.start
  measures "d1165" distance of P0 P3
  measures "d1166" distance of P0 P4
  measures "d1167" distance of P2 P6
  measures "d1168" distance of P6 P7
  measures "d1169" distance of L0 L3
  measures "d1170" distance of L6 L7
  measures "d1171" distance of L3 L9
  measures "d1172" distance of A17.centre L3
  measures "d1173" diameter of A17
  measures "d1174" distance of A17.centre L4
  measures "d1175" diameter of A20
  measures "d1176" distance of A20.centre L6
  measures "d1177" distance of A20.centre L3
  measures "d1600" radius of A34
  measures "d1601" radius of A35
  measures "d1602" radius of A36
  measures "d1603" radius of A37
  measures "d1604" radius of A38
  measures "d1605" radius of A39
  measures "d1606" radius of A40
  measures "d1607" radius of A41
  measures "d1696" diameter of A45
  measures "d1699" distance of L4 A47.centre
  measures "d1700" distance of L1 A49.centre
  measures "d1705" diameter of A73
  measures "d1707" distance of A80.centre L16
  measures "d1708" distance of L1 A93.centre
  measures "d1709" diameter of A97
  measures "d1710" diameter of A98
  measures "d1739" distance of L20.end L17.end
  measures "d1740" diameter of A107
  measures "d1741" radius of A106
  measures "d1742" radius of A105
sketch "Content (2)" plane through (0, 0, 0) normal (0, 0, 1) x (1, 0, 0) in component "Bottom"
  line L0 (-240, -184) -> (-240, -2) construction
  line L1 (-240, -2) -> (0, -2) construction
  line L2 (0, -184) -> (-240, -184) construction
  circle A0 centre (-139, -9) radius 1
  circle A1 centre (-15, -172) radius 1.75
  line L3 (0, -2) -> (0, -184) construction
  circle A2 centre (-120, -93.901) radius 1.05
  circle A3 centre (-225, -172) radius 1.75
  circle A4 centre (-225, -17) radius 1.75
  circle A5 centre (-139, -103) radius 1
  circle A6 centre (-15, -17) radius 1.75
  circle A7 centre (-233, -103) radius 1
  circle A8 centre (-233, -9) radius 1
  line L4 (1.75, 0) -> (22.5, 0) construction
  line L5 (0, 1.75) -> (0, 22.5) construction
  line L6 (0, -184) -> (-304.8, -184)
  circle A9 centre (-76.675, -120) radius 2
  circle A10 centre (-26.675, -120) radius 2
  circle A11 centre (-76.675, -151) radius 2
  circle A12 centre (-26.675, -151) radius 2
  line L7 (0, 425.6) -> (0, -184)
  circle A13 centre (-211.0542, -25.3538) radius 1.0005
  circle A14 centre (-157.9209, -25.3538) radius 1.0005
  circle A15 centre (-104.7876, -25.3538) radius 1.0005
  circle A16 centre (-51.6542, -25.3538) radius 1.0005
  circle A17 centre (-211.0542, -68.4205) radius 1.0005
  circle A18 centre (-157.9209, -68.4205) radius 1.0005
  circle A19 centre (-51.6542, -68.4205) radius 1.0005
  circle A20 centre (-211.0542, -111.4871) radius 1.0005
  circle A21 centre (-51.6542, -111.4871) radius 1.0005
  circle A22 centre (-211.0542, -154.5538) radius 1.0005
  circle A23 centre (-157.9209, -154.5538) radius 1.0005
  circle A24 centre (-104.7876, -154.5538) radius 1.0005
  circle A25 centre (-51.6542, -154.5538) radius 1.0005
  point P0 (-120, -93.901)
  point P1 (0, -2)
  dimension "d828" = 210
  dimension "d829" = -155
  dimension "d832" = 94
  dimension "d833" = -94
  dimension "d282" = 3.5
  dimension "d289" = 2
  dimension "d422" = 240
  dimension "d423" = 182
  dimension "d424" = 15
  dimension "d426" = 15
  dimension "d427" = 7
  dimension "d428" = 7
  dimension "d463" = 2.1
  dimension "d843" = 2
  dimension "d1634" = 4
  dimension "d1637" = 50
  dimension "d1638" = -31
  dimension "d1639" = 64
  dimension "d1640" = 26.675
  dimension "d1726" = 2.001
  dimension "d1729" = 159.4
  dimension "d1730" = -129.2
  constraint horizontal L2
  constraint perpendicular L0 L2
  constraint parallel L1 L2
  constraint coincident P0 A2.centre
  constraint coincident P1 L1.end
  constraint vertical L3
  constraint collinear L3 L5
  measures "d282" diameter of A4
  measures "d289" diameter of A8
  measures "d422" distance of P1 L0.end
  measures "d423" distance of L0.start L0.end
  measures "d424" distance of A4.centre L1
  measures "d426" distance of A4.centre L0
  measures "d427" distance of A8.centre L1
  measures "d428" distance of A8.centre L0
  measures "d463" diameter of A2
  measures "d843" distance of L1 L4
  measures "d1634" diameter of A9
  measures "d1639" distance of L2 A9.centre
  measures "d1640" distance of A12.centre L7
  measures "d1726" diameter of A13
sketch "Content (3)" plane through (0, 0, 0) normal (0, 0, 1) x (1, 0, 0) in component "Front"
  line L0 (242, 62) -> (2, 62) construction
  line L1 (2, 2) -> (242, 2) construction
  line L2 (2, 62) -> (2, 2) construction
  line L3 (242, 62) -> (242, 2) construction
  line L4 (0, 1.75) -> (0, 22.5) construction
  line L5 (1.75, 0) -> (22.5, 0) construction
  line L6 (39.175, 22.1755) -> (39.175, 46.6727) construction
  circle A0 centre (48.175, 16.175) radius 5
  circle A1 centre (48.175, 34.175) radius 9
  circle A2 centre (216.325, 32) radius 15
  circle A3 centre (216.325, 32) radius 1.5
  circle A4 centre (216.325, 56.5) radius 1.5
  circle A5 centre (216.325, 7.5) radius 1.5
  circle A6 centre (216.325, 32) radius 20.5 construction
  circle A7 centre (169.325, 32) radius 20.5 construction
  circle A8 centre (169.325, 32) radius 15
  circle A9 centre (169.325, 7.5) radius 1.5
  circle A10 centre (169.325, 32) radius 1.5
  circle A11 centre (169.325, 56.5) radius 1.5
  circle A12 centre (122.325, 32) radius 20.5 construction
  circle A13 centre (122.325, 32) radius 15
  circle A14 centre (122.325, 7.5) radius 1.5
  circle A15 centre (122.325, 32) radius 1.5
  circle A16 centre (122.325, 56.5) radius 1.5
  point P0 (1.401, 31.401)
  point P1 (47.095, 2)
  point P2 (242, 32)
  dimension "d492" = 240
  dimension "d493" = 60
  dimension "d1106" = 2
  dimension "d1400" = 2
  dimension "d1567" = 14.175
  dimension "d1568" = 10
  dimension "d1569" = 18
  dimension "d1570" = 18
  dimension "d1725" = 46.175
  dimension "d1746" = 30
  dimension "d1748" = 3
  dimension "d1751" = 0
  dimension "d1752" = -24.5
  dimension "d1753" = 41
  dimension "d1754" = 25.675
  dimension "d1757" = -47
  dimension "d1758" = 0
  constraint perpendicular L0 L2
  constraint perpendicular L0 L3
  constraint horizontal L1
  constraint vertical L6
  constraint vertical A0.centre A1.centre
  constraint tangent L6 A1
  constraint midpoint L3 P2
  constraint horizontal A2.centre P2
  constraint concentric A2 A3
  constraint concentric A2 A6
  measures "d492" distance of L0.end L0.start
  measures "d493" distance of L1.end L0.start
  measures "d1106" distance of L2 L4
  measures "d1400" distance of L1 L5
  measures "d1567" distance of L1 A0.centre
  measures "d1568" diameter of A0
  measures "d1569" diameter of A1
  measures "d1570" vertical distance of A0.centre A1.centre
  measures "d1725" distance of L2 A1.centre
  measures "d1746" diameter of A2
  measures "d1748" diameter of A3
  measures "d1753" diameter of A6
  measures "d1754" distance of L3 A2.centre